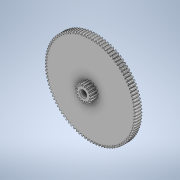
# Autodesk Inventor part: double_gear
Saved by Autodesk Inventor 2022.3 (Build 263350000, 350)
## iProperties
Created: 2022-06-10
Part Number: double_gear
Material: Generic
Document SubType Name: Modeling
Designer: Martijn
Density: 1 g/cm^3
Appearance: Default
Author: Martijn
Autodesk Inventor part; units mm, degrees
(part 1 of 3)
ref_plane "YZ Plane" through (0, 0, 0) normal (1, 0, 0) x (0, 1, 0)
ref_plane "XZ Plane" through (0, 0, 0) normal (0, 1, 0) x (-1, 0, 0)
ref_plane "XY Plane" through (0, 0, 0) normal (0, 0, 1) x (1, 0, 0)
sketch "Sketch1" plane through (0, 0, 0) normal (0, 0, 1) x (1, 0, 0)
  arc A0 (48.7229, -1.6254) -> (48.7288, -1.4372) centre (0, 0) ccw
  arc A1 (49.0225, -1.0633) -> (48.7288, -1.4372) centre (49.1286, -1.449) ccw
  spline S0 degree 3 poles (49.0225, -1.0633) (49.8054, -0.8336) (50.3699, -0.638) (50.9987, -0.3781) knots 0 0 0 0 1 1 1 1
  line L0 (49.0225, -1.0633) -> (49.8054, -0.8336) construction
  line L1 (49.8054, -0.8336) -> (50.3699, -0.638) construction
  line L2 (50.3699, -0.638) -> (50.9987, -0.3781) construction
  arc A2 (50.9987, -0.3781) -> (50.9987, 0.3781) centre (0, 0) ccw
  spline S1 degree 3 poles (50.9987, 0.3781) (50.3699, 0.638) (49.8054, 0.8336) (49.0225, 1.0633) knots 0 0 0 0 1 1 1 1
  line L3 (50.9987, 0.3781) -> (50.3699, 0.638) construction
  line L4 (50.3699, 0.638) -> (49.8054, 0.8336) construction
  line L5 (49.8054, 0.8336) -> (49.0225, 1.0633) construction
  arc A3 (48.7288, 1.4372) -> (49.0225, 1.0633) centre (49.1286, 1.449) ccw
  arc A4 (48.7288, 1.4372) -> (48.7229, 1.6254) centre (0, 0) ccw
  arc A5 (48.9926, 2.0169) -> (48.7229, 1.6254) centre (49.1227, 1.6387) ccw
  spline S2 degree 3 poles (48.9926, 2.0169) (49.7595, 2.2954) (50.3106, 2.526) (50.9218, 2.8249) knots 0 0 0 0 1 1 1 1
  line L6 (48.9926, 2.0169) -> (49.7595, 2.2954) construction
  line L7 (49.7595, 2.2954) -> (50.3106, 2.526) construction
  line L8 (50.3106, 2.526) -> (50.9218, 2.8249) construction
  arc A6 (50.9218, 2.8249) -> (50.8743, 3.5795) centre (0, 0) ccw
  spline S3 degree 3 poles (50.8743, 3.5795) (50.2305, 3.7995) (49.6548, 3.9592) (48.859, 4.1394) knots 0 0 0 0 1 1 1 1
  line L9 (50.8743, 3.5795) -> (50.2305, 3.7995) construction
  line L10 (50.2305, 3.7995) -> (49.6548, 3.9592) construction
  line L11 (49.6548, 3.9592) -> (48.859, 4.1394) construction
  arc A7 (48.5424, 4.4941) -> (48.859, 4.1394) centre (48.9407, 4.5309) ccw
  arc A8 (48.5424, 4.4941) -> (48.5247, 4.6815) centre (0, 0) ccw
  arc A9 (48.7692, 5.0892) -> (48.5247, 4.6815) centre (48.9228, 4.7199) ccw
  spline S4 degree 3 poles (48.7692, 5.0892) (49.5171, 5.4153) (50.0527, 5.68) (50.6439, 6.0168) knots 0 0 0 0 1 1 1 1
  line L12 (48.7692, 5.0892) -> (49.5171, 5.4153) construction
  line L13 (49.5171, 5.4153) -> (50.0527, 5.68) construction
  line L14 (50.0527, 5.68) -> (50.6439, 6.0168) construction
  arc A10 (50.6439, 6.0168) -> (50.5492, 6.7669) centre (0, 0) ccw
  spline S5 degree 3 poles (50.5492, 6.7669) (49.8928, 6.946) (49.3082, 7.0693) (48.5027, 7.1991) knots 0 0 0 0 1 1 1 1
  line L15 (50.5492, 6.7669) -> (49.8928, 6.946) construction
  line L16 (49.8928, 6.946) -> (49.3082, 7.0693) construction
  line L17 (49.3082, 7.0693) -> (48.5027, 7.1991) construction
  arc A11 (48.1644, 7.5332) -> (48.5027, 7.1991) centre (48.5596, 7.595) ccw
  arc A12 (48.1644, 7.5332) -> (48.135, 7.7191) centre (0, 0) ccw
  arc A13 (48.3535, 8.1414) -> (48.135, 7.7191) centre (48.5299, 7.7825) ccw
  spline S6 degree 3 poles (48.3535, 8.1414) (49.0794, 8.5138) (49.5973, 8.8117) (50.1662, 9.1848) knots 0 0 0 0 1 1 1 1
  line L18 (48.3535, 8.1414) -> (49.0794, 8.5138) construction
  line L19 (49.0794, 8.5138) -> (49.5973, 8.8117) construction
  line L20 (49.5973, 8.8117) -> (50.1662, 9.1848) construction
  arc A14 (50.1662, 9.1848) -> (50.0245, 9.9276) centre (0, 0) ccw
  spline S7 degree 3 poles (50.0245, 9.9276) (49.3582, 10.0651) (48.767, 10.1514) (47.955, 10.2304) knots 0 0 0 0 1 1 1 1
  line L21 (50.0245, 9.9276) -> (49.3582, 10.0651) construction
  line L22 (49.3582, 10.0651) -> (48.767, 10.1514) construction
  line L23 (48.767, 10.1514) -> (47.955, 10.2304) construction
  arc A15 (47.5964, 10.5426) -> (47.955, 10.2304) centre (47.9869, 10.6291) ccw
  arc A16 (47.5964, 10.5426) -> (47.5553, 10.7263) centre (0, 0) ccw
  arc A17 (47.7468, 11.1615) -> (47.5553, 10.7263) centre (47.9455, 10.8143) ccw
  spline S8 degree 3 poles (47.7468, 11.1615) (48.448, 11.5787) (48.9462, 11.9085) (49.4905, 12.3167) knots 0 0 0 0 1 1 1 1
  line L24 (47.7468, 11.1615) -> (48.448, 11.5787) construction
  line L25 (48.448, 11.5787) -> (48.9462, 11.9085) construction
  line L26 (48.9462, 11.9085) -> (49.4905, 12.3167) construction
  arc A18 (49.4905, 12.3167) -> (49.3024, 13.049) centre (0, 0) ccw
  spline S9 degree 3 poles (49.3024, 13.049) (48.6288, 13.1445) (48.0334, 13.1935) (47.218, 13.2213) knots 0 0 0 0 1 1 1 1
  line L27 (49.3024, 13.049) -> (48.6288, 13.1445) construction
  line L28 (48.6288, 13.1445) -> (48.0334, 13.1935) construction
  line L29 (48.0334, 13.1935) -> (47.218, 13.2213) construction
  arc A19 (46.8405, 13.5104) -> (47.218, 13.2213) centre (47.2248, 13.6213) ccw
  arc A20 (46.8405, 13.5104) -> (46.788, 13.6912) centre (0, 0) ccw
  arc A21 (46.9518, 14.1375) -> (46.788, 13.6912) centre (47.1719, 13.8035) ccw
  spline S10 degree 3 poles (46.9518, 14.1375) (47.6253, 14.5979) (48.1018, 14.9584) (48.6194, 15.3999) knots 0 0 0 0 1 1 1 1
  line L30 (46.9518, 14.1375) -> (47.6253, 14.5979) construction
  line L31 (47.6253, 14.5979) -> (48.1018, 14.9584) construction
  line L32 (48.1018, 14.9584) -> (48.6194, 15.3999) construction
  arc A22 (48.6194, 15.3999) -> (48.3858, 16.119) centre (0, 0) ccw
  spline S11 degree 3 poles (48.3858, 16.119) (47.7075, 16.172) (47.1102, 16.1835) (46.2946, 16.1601) knots 0 0 0 0 1 1 1 1
  line L33 (48.3858, 16.119) -> (47.7075, 16.172) construction
  line L34 (47.7075, 16.172) -> (47.1102, 16.1835) construction
  line L35 (47.1102, 16.1835) -> (46.2946, 16.1601) construction
  arc A23 (45.8997, 16.4249) -> (46.2946, 16.1601) centre (46.2763, 16.5596) ccw
  arc A24 (45.8997, 16.4249) -> (45.836, 16.602) centre (0, 0) ccw
  arc A25 (45.9714, 17.0578) -> (45.836, 16.602) centre (46.2121, 16.7382) ccw
  spline S12 degree 3 poles (45.9714, 17.0578) (46.6147, 17.5595) (47.0677, 17.9492) (47.5565, 18.4224) knots 0 0 0 0 1 1 1 1
  line L36 (45.9714, 17.0578) -> (46.6147, 17.5595) construction
  line L37 (46.6147, 17.5595) -> (47.0677, 17.9492) construction
  line L38 (47.0677, 17.9492) -> (47.5565, 18.4224) construction
  arc A26 (47.5565, 18.4224) -> (47.2782, 19.1254) centre (0, 0) ccw
  spline S13 degree 3 poles (47.2782, 19.1254) (46.5979, 19.1356) (46.001, 19.1096) (45.1886, 19.035) knots 0 0 0 0 1 1 1 1
  line L39 (47.2782, 19.1254) -> (46.5979, 19.1356) construction
  line L40 (46.5979, 19.1356) -> (46.001, 19.1096) construction
  line L41 (46.001, 19.1096) -> (45.1886, 19.035) construction
  arc A27 (44.7778, 19.2745) -> (45.1886, 19.035) centre (45.1452, 19.4327) ccw
  arc A28 (44.7778, 19.2745) -> (44.7031, 19.4473) centre (0, 0) ccw
  arc A29 (44.8097, 19.9107) -> (44.7031, 19.4473) centre (45.0699, 19.6069) ccw
  spline S14 degree 3 poles (44.8097, 19.9107) (45.4202, 20.4519) (45.8478, 20.8692) (46.3059, 21.3721) knots 0 0 0 0 1 1 1 1
  line L42 (44.8097, 19.9107) -> (45.4202, 20.4519) construction
  line L43 (45.4202, 20.4519) -> (45.8478, 20.8692) construction
  line L44 (45.8478, 20.8692) -> (46.3059, 21.3721) construction
  arc A30 (46.3059, 21.3721) -> (45.984, 22.0563) centre (0, 0) ccw
  spline S15 degree 3 poles (45.984, 22.0563) (45.3044, 22.0238) (44.7103, 21.9604) (43.9042, 21.8349) knots 0 0 0 0 1 1 1 1
  line L45 (45.984, 22.0563) -> (45.3044, 22.0238) construction
  line L46 (45.3044, 22.0238) -> (44.7103, 21.9604) construction
  line L47 (44.7103, 21.9604) -> (43.9042, 21.8349) construction
  arc A31 (43.4792, 22.0481) -> (43.9042, 21.8349) centre (43.836, 22.229) ccw
  arc A32 (43.4792, 22.0481) -> (43.3938, 22.2159) centre (0, 0) ccw
  arc A33 (43.471, 22.685) -> (43.3938, 22.2159) centre (43.7498, 22.3981) ccw
  spline S16 degree 3 poles (43.471, 22.685) (44.0464, 23.2635) (44.4469, 23.7068) (44.8726, 24.2375) knots 0 0 0 0 1 1 1 1
  line L48 (43.471, 22.685) -> (44.0464, 23.2635) construction
  line L49 (44.0464, 23.2635) -> (44.4469, 23.7068) construction
  line L50 (44.4469, 23.7068) -> (44.8726, 24.2375) construction
  arc A34 (44.8726, 24.2375) -> (44.5083, 24.9001) centre (0, 0) ccw
  spline S17 degree 3 poles (44.5083, 24.9001) (43.8322, 24.825) (43.2432, 24.7244) (42.4465, 24.5486) knots 0 0 0 0 1 1 1 1
  line L51 (44.5083, 24.9001) -> (43.8322, 24.825) construction
  line L52 (43.8322, 24.825) -> (43.2432, 24.7244) construction
  line L53 (43.2432, 24.7244) -> (42.4465, 24.5486) construction
  arc A35 (42.009, 24.7347) -> (42.4465, 24.5486) centre (42.3537, 24.9377) ccw
  arc A36 (42.009, 24.7347) -> (41.9132, 24.8967) centre (0, 0) ccw
  arc A37 (41.9609, 25.3698) -> (41.9132, 24.8967) centre (42.2571, 25.101) ccw
  spline S18 degree 3 poles (41.9609, 25.3698) (42.4987, 25.9832) (42.8706, 26.4509) (43.2622, 27.0072) knots 0 0 0 0 1 1 1 1
  line L54 (41.9609, 25.3698) -> (42.4987, 25.9832) construction
  line L55 (42.4987, 25.9832) -> (42.8706, 26.4509) construction
  line L56 (42.8706, 26.4509) -> (43.2622, 27.0072) construction
  arc A38 (43.2622, 27.0072) -> (42.857, 27.6457) centre (0, 0) ccw
  spline S19 degree 3 poles (42.857, 27.6457) (42.1869, 27.5283) (41.6054, 27.3909) (40.8213, 27.1654) knots 0 0 0 0 1 1 1 1
  line L57 (42.857, 27.6457) -> (42.1869, 27.5283) construction
  line L58 (42.1869, 27.5283) -> (41.6054, 27.3909) construction
  line L59 (41.6054, 27.3909) -> (40.8213, 27.1654) construction
  arc A39 (40.373, 27.3237) -> (40.8213, 27.1654) centre (40.7043, 27.5479) ccw
  arc A40 (40.373, 27.3237) -> (40.2672, 27.4794) centre (0, 0) ccw
  arc A41 (40.2851, 27.9545) -> (40.2672, 27.4794) centre (40.5976, 27.7048) ccw
  spline S20 degree 3 poles (40.2851, 27.9545) (40.7834, 28.6005) (41.1252, 29.0905) (41.481, 29.6704) knots 0 0 0 0 1 1 1 1
  line L60 (40.2851, 27.9545) -> (40.7834, 28.6005) construction
  line L61 (40.7834, 28.6005) -> (41.1252, 29.0905) construction
  line L62 (41.1252, 29.0905) -> (41.481, 29.6704) construction
  arc A42 (41.481, 29.6704) -> (41.0366, 30.2821) centre (0, 0) ccw
  spline S21 degree 3 poles (41.0366, 30.2821) (40.3751, 30.1229) (39.8034, 29.9493) (39.0351, 29.675) knots 0 0 0 0 1 1 1 1
  line L63 (41.0366, 30.2821) -> (40.3751, 30.1229) construction
  line L64 (40.3751, 30.1229) -> (39.8034, 29.9493) construction
  line L65 (39.8034, 29.9493) -> (39.0351, 29.675) construction
  arc A43 (38.5777, 29.8048) -> (39.0351, 29.675) centre (38.8942, 30.0493) ccw
  arc A44 (38.5777, 29.8048) -> (38.4623, 29.9535) centre (0, 0) ccw
  arc A45 (38.4503, 30.4288) -> (38.4623, 29.9535) centre (38.7779, 30.1993) ccw
  spline S22 degree 3 poles (38.4503, 30.4288) (38.9071, 31.1049) (39.2174, 31.6154) (39.5361, 32.2165) knots 0 0 0 0 1 1 1 1
  line L66 (38.4503, 30.4288) -> (38.9071, 31.1049) construction
  line L67 (38.9071, 31.1049) -> (39.2174, 31.6154) construction
  line L68 (39.2174, 31.6154) -> (39.5361, 32.2165) construction
  arc A46 (39.5361, 32.2165) -> (39.0542, 32.7991) centre (0, 0) ccw
  spline S23 degree 3 poles (39.0542, 32.7991) (38.404, 32.5986) (37.8444, 32.3894) (37.0947, 32.0674) knots 0 0 0 0 1 1 1 1
  line L69 (39.0542, 32.7991) -> (38.404, 32.5986) construction
  line L70 (38.404, 32.5986) -> (37.8444, 32.3894) construction
  line L71 (37.8444, 32.3894) -> (37.0947, 32.0674) construction
  arc A47 (36.6301, 32.1683) -> (37.0947, 32.0674) centre (36.9306, 32.4322) ccw
  arc A48 (36.6301, 32.1683) -> (36.5056, 32.3095) centre (0, 0) ccw
  arc A49 (36.4638, 32.7831) -> (36.5056, 32.3095) centre (36.8051, 32.5746) ccw
  spline S24 degree 3 poles (36.4638, 32.7831) (36.8772, 33.4865) (37.1549, 34.0155) (37.4352, 34.6354) knots 0 0 0 0 1 1 1 1
  line L72 (36.4638, 32.7831) -> (36.8772, 33.4865) construction
  line L73 (36.8772, 33.4865) -> (37.1549, 34.0155) construction
  line L74 (37.1549, 34.0155) -> (37.4352, 34.6354) construction
  arc A50 (37.4352, 34.6354) -> (36.9176, 35.1866) centre (0, 0) ccw
  spline S25 degree 3 poles (36.9176, 35.1866) (36.2814, 34.9457) (35.7359, 34.7018) (35.008, 34.3334) knots 0 0 0 0 1 1 1 1
  line L75 (36.9176, 35.1866) -> (36.2814, 34.9457) construction
  line L76 (36.2814, 34.9457) -> (35.7359, 34.7018) construction
  line L77 (35.7359, 34.7018) -> (35.008, 34.3334) construction
  arc A51 (34.538, 34.4048) -> (35.008, 34.3334) centre (34.8213, 34.6871) ccw
  arc A52 (34.538, 34.4048) -> (34.4048, 34.538) centre (0, 0) ccw
  arc A53 (34.3334, 35.008) -> (34.4048, 34.538) centre (34.6871, 34.8213) ccw
  spline S26 degree 3 poles (34.3334, 35.008) (34.7018, 35.7359) (34.9457, 36.2814) (35.1866, 36.9176) knots 0 0 0 0 1 1 1 1
  line L78 (34.3334, 35.008) -> (34.7018, 35.7359) construction
  line L79 (34.7018, 35.7359) -> (34.9457, 36.2814) construction
  line L80 (34.9457, 36.2814) -> (35.1866, 36.9176) construction
  arc A54 (35.1866, 36.9176) -> (34.6354, 37.4352) centre (0, 0) ccw
  spline S27 degree 3 poles (34.6354, 37.4352) (34.0155, 37.1549) (33.4865, 36.8772) (32.7831, 36.4638) knots 0 0 0 0 1 1 1 1
  line L81 (34.6354, 37.4352) -> (34.0155, 37.1549) construction
  line L82 (34.0155, 37.1549) -> (33.4865, 36.8772) construction
  line L83 (33.4865, 36.8772) -> (32.7831, 36.4638) construction
  arc A55 (32.3095, 36.5056) -> (32.7831, 36.4638) centre (32.5746, 36.8051) ccw
  arc A56 (32.3095, 36.5056) -> (32.1683, 36.6301) centre (0, 0) ccw
  arc A57 (32.0674, 37.0947) -> (32.1683, 36.6301) centre (32.4322, 36.9306) ccw
  spline S28 degree 3 poles (32.0674, 37.0947) (32.3894, 37.8444) (32.5986, 38.404) (32.7991, 39.0542) knots 0 0 0 0 1 1 1 1
  line L84 (32.0674, 37.0947) -> (32.3894, 37.8444) construction
  line L85 (32.3894, 37.8444) -> (32.5986, 38.404) construction
  line L86 (32.5986, 38.404) -> (32.7991, 39.0542) construction
  arc A58 (32.7991, 39.0542) -> (32.2165, 39.5361) centre (0, 0) ccw
  spline S29 degree 3 poles (32.2165, 39.5361) (31.6154, 39.2174) (31.1049, 38.9071) (30.4288, 38.4503) knots 0 0 0 0 1 1 1 1
  line L87 (32.2165, 39.5361) -> (31.6154, 39.2174) construction
  line L88 (31.6154, 39.2174) -> (31.1049, 38.9071) construction
  line L89 (31.1049, 38.9071) -> (30.4288, 38.4503) construction
  arc A59 (29.9535, 38.4623) -> (30.4288, 38.4503) centre (30.1993, 38.7779) ccw
  arc A60 (29.9535, 38.4623) -> (29.8048, 38.5777) centre (0, 0) ccw
  arc A61 (29.675, 39.0351) -> (29.8048, 38.5777) centre (30.0493, 38.8942) ccw
  spline S30 degree 3 poles (29.675, 39.0351) (29.9493, 39.8034) (30.1229, 40.3751) (30.2821, 41.0366) knots 0 0 0 0 1 1 1 1
  line L90 (29.675, 39.0351) -> (29.9493, 39.8034) construction
  line L91 (29.9493, 39.8034) -> (30.1229, 40.3751) construction
  line L92 (30.1229, 40.3751) -> (30.2821, 41.0366) construction
  arc A62 (30.2821, 41.0366) -> (29.6704, 41.481) centre (0, 0) ccw
  spline S31 degree 3 poles (29.6704, 41.481) (29.0905, 41.1252) (28.6005, 40.7834) (27.9545, 40.2851) knots 0 0 0 0 1 1 1 1
  line L93 (29.6704, 41.481) -> (29.0905, 41.1252) construction
  line L94 (29.0905, 41.1252) -> (28.6005, 40.7834) construction
  line L95 (28.6005, 40.7834) -> (27.9545, 40.2851) construction
  arc A63 (27.4794, 40.2672) -> (27.9545, 40.2851) centre (27.7048, 40.5976) ccw
  arc A64 (27.4794, 40.2672) -> (27.3237, 40.373) centre (0, 0) ccw
  arc A65 (27.1654, 40.8213) -> (27.3237, 40.373) centre (27.5479, 40.7043) ccw
  spline S32 degree 3 poles (27.1654, 40.8213) (27.3909, 41.6054) (27.5283, 42.1869) (27.6457, 42.857) knots 0 0 0 0 1 1 1 1
  line L96 (27.1654, 40.8213) -> (27.3909, 41.6054) construction
  line L97 (27.3909, 41.6054) -> (27.5283, 42.1869) construction
  line L98 (27.5283, 42.1869) -> (27.6457, 42.857) construction
  arc A66 (27.6457, 42.857) -> (27.0072, 43.2622) centre (0, 0) ccw
  spline S33 degree 3 poles (27.0072, 43.2622) (26.4509, 42.8706) (25.9832, 42.4987) (25.3698, 41.9609) knots 0 0 0 0 1 1 1 1
  line L99 (27.0072, 43.2622) -> (26.4509, 42.8706) construction
  line L100 (26.4509, 42.8706) -> (25.9832, 42.4987) construction
  line L101 (25.9832, 42.4987) -> (25.3698, 41.9609) construction
  arc A67 (24.8967, 41.9132) -> (25.3698, 41.9609) centre (25.101, 42.2571) ccw
  arc A68 (24.8967, 41.9132) -> (24.7347, 42.009) centre (0, 0) ccw
  arc A69 (24.5486, 42.4465) -> (24.7347, 42.009) centre (24.9377, 42.3537) ccw
  spline S34 degree 3 poles (24.5486, 42.4465) (24.7244, 43.2432) (24.825, 43.8322) (24.9001, 44.5083) knots 0 0 0 0 1 1 1 1
  line L102 (24.5486, 42.4465) -> (24.7244, 43.2432) construction
  line L103 (24.7244, 43.2432) -> (24.825, 43.8322) construction
  line L104 (24.825, 43.8322) -> (24.9001, 44.5083) construction
  arc A70 (24.9001, 44.5083) -> (24.2375, 44.8726) centre (0, 0) ccw
  spline S35 degree 3 poles (24.2375, 44.8726) (23.7068, 44.4469) (23.2635, 44.0464) (22.685, 43.471) knots 0 0 0 0 1 1 1 1
  line L105 (24.2375, 44.8726) -> (23.7068, 44.4469) construction
  line L106 (23.7068, 44.4469) -> (23.2635, 44.0464) construction
  line L107 (23.2635, 44.0464) -> (22.685, 43.471) construction
  arc A71 (22.2159, 43.3938) -> (22.685, 43.471) centre (22.3981, 43.7498) ccw
  arc A72 (22.2159, 43.3938) -> (22.0481, 43.4792) centre (0, 0) ccw
  arc A73 (21.8349, 43.9042) -> (22.0481, 43.4792) centre (22.229, 43.836) ccw
  spline S36 degree 3 poles (21.8349, 43.9042) (21.9604, 44.7103) (22.0238, 45.3044) (22.0563, 45.984) knots 0 0 0 0 1 1 1 1
  line L108 (21.8349, 43.9042) -> (21.9604, 44.7103) construction
  line L109 (21.9604, 44.7103) -> (22.0238, 45.3044) construction
  line L110 (22.0238, 45.3044) -> (22.0563, 45.984) construction
  arc A74 (22.0563, 45.984) -> (21.3721, 46.3059) centre (0, 0) ccw
  spline S37 degree 3 poles (21.3721, 46.3059) (20.8692, 45.8478) (20.4519, 45.4202) (19.9107, 44.8097) knots 0 0 0 0 1 1 1 1
  line L111 (21.3721, 46.3059) -> (20.8692, 45.8478) construction
  line L112 (20.8692, 45.8478) -> (20.4519, 45.4202) construction
  line L113 (20.4519, 45.4202) -> (19.9107, 44.8097) construction
  arc A75 (19.4473, 44.7031) -> (19.9107, 44.8097) centre (19.6069, 45.0699) ccw
  arc A76 (19.4473, 44.7031) -> (19.2745, 44.7778) centre (0, 0) ccw
  arc A77 (19.035, 45.1886) -> (19.2745, 44.7778) centre (19.4327, 45.1452) ccw
  spline S38 degree 3 poles (19.035, 45.1886) (19.1096, 46.001) (19.1356, 46.5979) (19.1254, 47.2782) knots 0 0 0 0 1 1 1 1
  line L114 (19.035, 45.1886) -> (19.1096, 46.001) construction
  line L115 (19.1096, 46.001) -> (19.1356, 46.5979) construction
  line L116 (19.1356, 46.5979) -> (19.1254, 47.2782) construction
  arc A78 (19.1254, 47.2782) -> (18.4224, 47.5565) centre (0, 0) ccw
  spline S39 degree 3 poles (18.4224, 47.5565) (17.9492, 47.0677) (17.5595, 46.6147) (17.0578, 45.9714) knots 0 0 0 0 1 1 1 1
  line L117 (18.4224, 47.5565) -> (17.9492, 47.0677) construction
  line L118 (17.9492, 47.0677) -> (17.5595, 46.6147) construction
  line L119 (17.5595, 46.6147) -> (17.0578, 45.9714) construction
  arc A79 (16.602, 45.836) -> (17.0578, 45.9714) centre (16.7382, 46.2121) ccw
  arc A80 (16.602, 45.836) -> (16.4249, 45.8997) centre (0, 0) ccw
  arc A81 (16.1601, 46.2946) -> (16.4249, 45.8997) centre (16.5596, 46.2763) ccw
  spline S40 degree 3 poles (16.1601, 46.2946) (16.1835, 47.1102) (16.172, 47.7075) (16.119, 48.3858) knots 0 0 0 0 1 1 1 1
  line L120 (16.1601, 46.2946) -> (16.1835, 47.1102) construction
  line L121 (16.1835, 47.1102) -> (16.172, 47.7075) construction
  line L122 (16.172, 47.7075) -> (16.119, 48.3858) construction
  arc A82 (16.119, 48.3858) -> (15.3999, 48.6194) centre (0, 0) ccw
  spline S41 degree 3 poles (15.3999, 48.6194) (14.9584, 48.1018) (14.5979, 47.6253) (14.1375, 46.9518) knots 0 0 0 0 1 1 1 1
  line L123 (15.3999, 48.6194) -> (14.9584, 48.1018) construction
  line L124 (14.9584, 48.1018) -> (14.5979, 47.6253) construction
  line L125 (14.5979, 47.6253) -> (14.1375, 46.9518) construction
  arc A83 (13.6912, 46.788) -> (14.1375, 46.9518) centre (13.8035, 47.1719) ccw
  arc A84 (13.6912, 46.788) -> (13.5104, 46.8405) centre (0, 0) ccw
  arc A85 (13.2213, 47.218) -> (13.5104, 46.8405) centre (13.6213, 47.2248) ccw
  spline S42 degree 3 poles (13.2213, 47.218) (13.1935, 48.0334) (13.1445, 48.6288) (13.049, 49.3024) knots 0 0 0 0 1 1 1 1
  line L126 (13.2213, 47.218) -> (13.1935, 48.0334) construction
  line L127 (13.1935, 48.0334) -> (13.1445, 48.6288) construction
  line L128 (13.1445, 48.6288) -> (13.049, 49.3024) construction
  arc A86 (13.049, 49.3024) -> (12.3167, 49.4905) centre (0, 0) ccw
  spline S43 degree 3 poles (12.3167, 49.4905) (11.9085, 48.9462) (11.5787, 48.448) (11.1615, 47.7468) knots 0 0 0 0 1 1 1 1
  line L129 (12.3167, 49.4905) -> (11.9085, 48.9462) construction
  line L130 (11.9085, 48.9462) -> (11.5787, 48.448) construction
  line L131 (11.5787, 48.448) -> (11.1615, 47.7468) construction
  arc A87 (10.7263, 47.5553) -> (11.1615, 47.7468) centre (10.8143, 47.9455) ccw
  arc A88 (10.7263, 47.5553) -> (10.5426, 47.5964) centre (0, 0) ccw
  arc A89 (10.2304, 47.955) -> (10.5426, 47.5964) centre (10.6291, 47.9869) ccw
  spline S44 degree 3 poles (10.2304, 47.955) (10.1514, 48.767) (10.0651, 49.3582) (9.9276, 50.0245) knots 0 0 0 0 1 1 1 1
  line L132 (10.2304, 47.955) -> (10.1514, 48.767) construction
  line L133 (10.1514, 48.767) -> (10.0651, 49.3582) construction
  line L134 (10.0651, 49.3582) -> (9.9276, 50.0245) construction
  arc A90 (9.9276, 50.0245) -> (9.1848, 50.1662) centre (0, 0) ccw
  spline S45 degree 3 poles (9.1848, 50.1662) (8.8117, 49.5973) (8.5138, 49.0794) (8.1414, 48.3535) knots 0 0 0 0 1 1 1 1
  line L135 (9.1848, 50.1662) -> (8.8117, 49.5973) construction
  line L136 (8.8117, 49.5973) -> (8.5138, 49.0794) construction
  line L137 (8.5138, 49.0794) -> (8.1414, 48.3535) construction
  arc A91 (7.7191, 48.135) -> (8.1414, 48.3535) centre (7.7825, 48.5299) ccw
  arc A92 (7.7191, 48.135) -> (7.5332, 48.1644) centre (0, 0) ccw
  arc A93 (7.1991, 48.5027) -> (7.5332, 48.1644) centre (7.595, 48.5596) ccw
  spline S46 degree 3 poles (7.1991, 48.5027) (7.0693, 49.3082) (6.946, 49.8928) (6.7669, 50.5492) knots 0 0 0 0 1 1 1 1
  line L138 (7.1991, 48.5027) -> (7.0693, 49.3082) construction
  line L139 (7.0693, 49.3082) -> (6.946, 49.8928) construction
  line L140 (6.946, 49.8928) -> (6.7669, 50.5492) construction
  arc A94 (6.7669, 50.5492) -> (6.0168, 50.6439) centre (0, 0) ccw
  spline S47 degree 3 poles (6.0168, 50.6439) (5.68, 50.0527) (5.4153, 49.5171) (5.0892, 48.7692) knots 0 0 0 0 1 1 1 1
  line L141 (6.0168, 50.6439) -> (5.68, 50.0527) construction
  line L142 (5.68, 50.0527) -> (5.4153, 49.5171) construction
  line L143 (5.4153, 49.5171) -> (5.0892, 48.7692) construction
  arc A95 (4.6815, 48.5247) -> (5.0892, 48.7692) centre (4.7199, 48.9228) ccw
  arc A96 (4.6815, 48.5247) -> (4.4941, 48.5424) centre (0, 0) ccw
  arc A97 (4.1394, 48.859) -> (4.4941, 48.5424) centre (4.5309, 48.9407) ccw
  spline S48 degree 3 poles (4.1394, 48.859) (3.9592, 49.6548) (3.7995, 50.2305) (3.5795, 50.8743) knots 0 0 0 0 1 1 1 1
  line L144 (4.1394, 48.859) -> (3.9592, 49.6548) construction
  line L145 (3.9592, 49.6548) -> (3.7995, 50.2305) construction
  line L146 (3.7995, 50.2305) -> (3.5795, 50.8743) construction
  arc A98 (3.5795, 50.8743) -> (2.8249, 50.9218) centre (0, 0) ccw
  spline S49 degree 3 poles (2.8249, 50.9218) (2.526, 50.3106) (2.2954, 49.7595) (2.0169, 48.9926) knots 0 0 0 0 1 1 1 1
  line L147 (2.8249, 50.9218) -> (2.526, 50.3106) construction
  line L148 (2.526, 50.3106) -> (2.2954, 49.7595) construction
  line L149 (2.2954, 49.7595) -> (2.0169, 48.9926) construction
  arc A99 (1.6254, 48.7229) -> (2.0169, 48.9926) centre (1.6387, 49.1227) ccw
  arc A100 (1.6254, 48.7229) -> (1.4372, 48.7288) centre (0, 0) ccw
  arc A101 (1.0633, 49.0225) -> (1.4372, 48.7288) centre (1.449, 49.1286) ccw
  spline S50 degree 3 poles (1.0633, 49.0225) (0.8336, 49.8054) (0.638, 50.3699) (0.3781, 50.9987) knots 0 0 0 0 1 1 1 1
  line L150 (1.0633, 49.0225) -> (0.8336, 49.8054) construction
  line L151 (0.8336, 49.8054) -> (0.638, 50.3699) construction
  line L152 (0.638, 50.3699) -> (0.3781, 50.9987) construction
  arc A102 (0.3781, 50.9987) -> (-0.3781, 50.9987) centre (0, 0) ccw
  spline S51 degree 3 poles (-0.3781, 50.9987) (-0.638, 50.3699) (-0.8336, 49.8054) (-1.0633, 49.0225) knots 0 0 0 0 1 1 1 1
  line L153 (-0.3781, 50.9987) -> (-0.638, 50.3699) construction
  line L154 (-0.638, 50.3699) -> (-0.8336, 49.8054) construction
  line L155 (-0.8336, 49.8054) -> (-1.0633, 49.0225) construction
  arc A103 (-1.4372, 48.7288) -> (-1.0633, 49.0225) centre (-1.449, 49.1286) ccw
  arc A104 (-1.4372, 48.7288) -> (-1.6254, 48.7229) centre (0, 0) ccw
  arc A105 (-2.0169, 48.9926) -> (-1.6254, 48.7229) centre (-1.6387, 49.1227) ccw
  spline S52 degree 3 poles (-2.0169, 48.9926) (-2.2954, 49.7595) (-2.526, 50.3106) (-2.8249, 50.9218) knots 0 0 0 0 1 1 1 1
  line L156 (-2.0169, 48.9926) -> (-2.2954, 49.7595) construction
  line L157 (-2.2954, 49.7595) -> (-2.526, 50.3106) construction
  line L158 (-2.526, 50.3106) -> (-2.8249, 50.9218) construction
  arc A106 (-2.8249, 50.9218) -> (-3.5795, 50.8743) centre (0, 0) ccw
  spline S53 degree 3 poles (-3.5795, 50.8743) (-3.7995, 50.2305) (-3.9592, 49.6548) (-4.1394, 48.859) knots 0 0 0 0 1 1 1 1
  line L159 (-3.5795, 50.8743) -> (-3.7995, 50.2305) construction
  line L160 (-3.7995, 50.2305) -> (-3.9592, 49.6548) construction
  line L161 (-3.9592, 49.6548) -> (-4.1394, 48.859) construction
  arc A107 (-4.4941, 48.5424) -> (-4.1394, 48.859) centre (-4.5309, 48.9407) ccw
  arc A108 (-4.4941, 48.5424) -> (-4.6815, 48.5247) centre (0, 0) ccw
  arc A109 (-5.0892, 48.7692) -> (-4.6815, 48.5247) centre (-4.7199, 48.9228) ccw
  spline S54 degree 3 poles (-5.0892, 48.7692) (-5.4153, 49.5171) (-5.68, 50.0527) (-6.0168, 50.6439) knots 0 0 0 0 1 1 1 1
  line L162 (-5.0892, 48.7692) -> (-5.4153, 49.5171) construction
  line L163 (-5.4153, 49.5171) -> (-5.68, 50.0527) construction
  line L164 (-5.68, 50.0527) -> (-6.0168, 50.6439) construction
  arc A110 (-6.0168, 50.6439) -> (-6.7669, 50.5492) centre (0, 0) ccw
  spline S55 degree 3 poles (-6.7669, 50.5492) (-6.946, 49.8928) (-7.0693, 49.3082) (-7.1991, 48.5027) knots 0 0 0 0 1 1 1 1
  line L165 (-6.7669, 50.5492) -> (-6.946, 49.8928) construction
  line L166 (-6.946, 49.8928) -> (-7.0693, 49.3082) construction
  line L167 (-7.0693, 49.3082) -> (-7.1991, 48.5027) construction
  arc A111 (-7.5332, 48.1644) -> (-7.1991, 48.5027) centre (-7.595, 48.5596) ccw
  arc A112 (-7.5332, 48.1644) -> (-7.7191, 48.135) centre (0, 0) ccw
  arc A113 (-8.1414, 48.3535) -> (-7.7191, 48.135) centre (-7.7825, 48.5299) ccw
  spline S56 degree 3 poles (-8.1414, 48.3535) (-8.5138, 49.0794) (-8.8117, 49.5973) (-9.1848, 50.1662) knots 0 0 0 0 1 1 1 1
  line L168 (-8.1414, 48.3535) -> (-8.5138, 49.0794) construction
  line L169 (-8.5138, 49.0794) -> (-8.8117, 49.5973) construction
  line L170 (-8.8117, 49.5973) -> (-9.1848, 50.1662) construction
  arc A114 (-9.1848, 50.1662) -> (-9.9276, 50.0245) centre (0, 0) ccw
  spline S57 degree 3 poles (-9.9276, 50.0245) (-10.0651, 49.3582) (-10.1514, 48.767) (-10.2304, 47.955) knots 0 0 0 0 1 1 1 1
  line L171 (-9.9276, 50.0245) -> (-10.0651, 49.3582) construction
  line L172 (-10.0651, 49.3582) -> (-10.1514, 48.767) construction
  line L173 (-10.1514, 48.767) -> (-10.2304, 47.955) construction
  arc A115 (-10.5426, 47.5964) -> (-10.2304, 47.955) centre (-10.6291, 47.9869) ccw
  arc A116 (-10.5426, 47.5964) -> (-10.7263, 47.5553) centre (0, 0) ccw
  arc A117 (-11.1615, 47.7468) -> (-10.7263, 47.5553) centre (-10.8143, 47.9455) ccw
  spline S58 degree 3 poles (-11.1615, 47.7468) (-11.5787, 48.448) (-11.9085, 48.9462) (-12.3167, 49.4905) knots 0 0 0 0 1 1 1 1
  line L174 (-11.1615, 47.7468) -> (-11.5787, 48.448) construction
  line L175 (-11.5787, 48.448) -> (-11.9085, 48.9462) construction
  line L176 (-11.9085, 48.9462) -> (-12.3167, 49.4905) construction
  arc A118 (-12.3167, 49.4905) -> (-13.049, 49.3024) centre (0, 0) ccw
  spline S59 degree 3 poles (-13.049, 49.3024) (-13.1445, 48.6288) (-13.1935, 48.0334) (-13.2213, 47.218) knots 0 0 0 0 1 1 1 1
  line L177 (-13.049, 49.3024) -> (-13.1445, 48.6288) construction
  line L178 (-13.1445, 48.6288) -> (-13.1935, 48.0334) construction
  line L179 (-13.1935, 48.0334) -> (-13.2213, 47.218) construction
  arc A119 (-13.5104, 46.8405) -> (-13.2213, 47.218) centre (-13.6213, 47.2248) ccw
  arc A120 (-13.5104, 46.8405) -> (-13.6912, 46.788) centre (0, 0) ccw
  arc A121 (-14.1375, 46.9518) -> (-13.6912, 46.788) centre (-13.8035, 47.1719) ccw
  spline S60 degree 3 poles (-14.1375, 46.9518) (-14.5979, 47.6253) (-14.9584, 48.1018) (-15.3999, 48.6194) knots 0 0 0 0 1 1 1 1
  line L180 (-14.1375, 46.9518) -> (-14.5979, 47.6253) construction
  line L181 (-14.5979, 47.6253) -> (-14.9584, 48.1018) construction
  line L182 (-14.9584, 48.1018) -> (-15.3999, 48.6194) construction
  arc A122 (-15.3999, 48.6194) -> (-16.119, 48.3858) centre (0, 0) ccw
  spline S61 degree 3 poles (-16.119, 48.3858) (-16.172, 47.7075) (-16.1835, 47.1102) (-16.1601, 46.2946) knots 0 0 0 0 1 1 1 1
  line L183 (-16.119, 48.3858) -> (-16.172, 47.7075) construction
  line L184 (-16.172, 47.7075) -> (-16.1835, 47.1102) construction
  line L185 (-16.1835, 47.1102) -> (-16.1601, 46.2946) construction
  arc A123 (-16.4249, 45.8997) -> (-16.1601, 46.2946) centre (-16.5596, 46.2763) ccw
  arc A124 (-16.4249, 45.8997) -> (-16.602, 45.836) centre (0, 0) ccw
  arc A125 (-17.0578, 45.9714) -> (-16.602, 45.836) centre (-16.7382, 46.2121) ccw
  spline S62 degree 3 poles (-17.0578, 45.9714) (-17.5595, 46.6147) (-17.9492, 47.0677) (-18.4224, 47.5565) knots 0 0 0 0 1 1 1 1
  line L186 (-17.0578, 45.9714) -> (-17.5595, 46.6147) construction
  line L187 (-17.5595, 46.6147) -> (-17.9492, 47.0677) construction
  line L188 (-17.9492, 47.0677) -> (-18.4224, 47.5565) construction
  arc A126 (-18.4224, 47.5565) -> (-19.1254, 47.2782) centre (0, 0) ccw
  spline S63 degree 3 poles (-19.1254, 47.2782) (-19.1356, 46.5979) (-19.1096, 46.001) (-19.035, 45.1886) knots 0 0 0 0 1 1 1 1
  line L189 (-19.1254, 47.2782) -> (-19.1356, 46.5979) construction
  line L190 (-19.1356, 46.5979) -> (-19.1096, 46.001) construction
  line L191 (-19.1096, 46.001) -> (-19.035, 45.1886) construction
  arc A127 (-19.2745, 44.7778) -> (-19.035, 45.1886) centre (-19.4327, 45.1452) ccw
  arc A128 (-19.2745, 44.7778) -> (-19.4473, 44.7031) centre (0, 0) ccw
  arc A129 (-19.9107, 44.8097) -> (-19.4473, 44.7031) centre (-19.6069, 45.0699) ccw
  spline S64 degree 3 poles (-19.9107, 44.8097) (-20.4519, 45.4202) (-20.8692, 45.8478) (-21.3721, 46.3059) knots 0 0 0 0 1 1 1 1
  line L192 (-19.9107, 44.8097) -> (-20.4519, 45.4202) construction
  line L193 (-20.4519, 45.4202) -> (-20.8692, 45.8478) construction
  line L194 (-20.8692, 45.8478) -> (-21.3721, 46.3059) construction
  arc A130 (-21.3721, 46.3059) -> (-22.0563, 45.984) centre (0, 0) ccw
  spline S65 degree 3 poles (-22.0563, 45.984) (-22.0238, 45.3044) (-21.9604, 44.7103) (-21.8349, 43.9042) knots 0 0 0 0 1 1 1 1
  line L195 (-22.0563, 45.984) -> (-22.0238, 45.3044) construction
  line L196 (-22.0238, 45.3044) -> (-21.9604, 44.7103) construction
  line L197 (-21.9604, 44.7103) -> (-21.8349, 43.9042) construction
  arc A131 (-22.0481, 43.4792) -> (-21.8349, 43.9042) centre (-22.229, 43.836) ccw
  arc A132 (-22.0481, 43.4792) -> (-22.2159, 43.3938) centre (0, 0) ccw
  arc A133 (-22.685, 43.471) -> (-22.2159, 43.3938) centre (-22.3981, 43.7498) ccw
  spline S66 degree 3 poles (-22.685, 43.471) (-23.2635, 44.0464) (-23.7068, 44.4469) (-24.2375, 44.8726) knots 0 0 0 0 1 1 1 1
  line L198 (-22.685, 43.471) -> (-23.2635, 44.0464) construction
  line L199 (-23.2635, 44.0464) -> (-23.7068, 44.4469) construction
  line L200 (-23.7068, 44.4469) -> (-24.2375, 44.8726) construction
  arc A134 (-24.2375, 44.8726) -> (-24.9001, 44.5083) centre (0, 0) ccw
  spline S67 degree 3 poles (-24.9001, 44.5083) (-24.825, 43.8322) (-24.7244, 43.2432) (-24.5486, 42.4465) knots 0 0 0 0 1 1 1 1
  line L201 (-24.9001, 44.5083) -> (-24.825, 43.8322) construction
  line L202 (-24.825, 43.8322) -> (-24.7244, 43.2432) construction
  line L203 (-24.7244, 43.2432) -> (-24.5486, 42.4465) construction
  arc A135 (-24.7347, 42.009) -> (-24.5486, 42.4465) centre (-24.9377, 42.3537) ccw
  arc A136 (-24.7347, 42.009) -> (-24.8967, 41.9132) centre (0, 0) ccw
  arc A137 (-25.3698, 41.9609) -> (-24.8967, 41.9132) centre (-25.101, 42.2571) ccw
  spline S68 degree 3 poles (-25.3698, 41.9609) (-25.9832, 42.4987) (-26.4509, 42.8706) (-27.0072, 43.2622) knots 0 0 0 0 1 1 1 1
  line L204 (-25.3698, 41.9609) -> (-25.9832, 42.4987) construction
  line L205 (-25.9832, 42.4987) -> (-26.4509, 42.8706) construction
  line L206 (-26.4509, 42.8706) -> (-27.0072, 43.2622) construction
  arc A138 (-27.0072, 43.2622) -> (-27.6457, 42.857) centre (0, 0) ccw
  spline S69 degree 3 poles (-27.6457, 42.857) (-27.5283, 42.1869) (-27.3909, 41.6054) (-27.1654, 40.8213) knots 0 0 0 0 1 1 1 1
  line L207 (-27.6457, 42.857) -> (-27.5283, 42.1869) construction
  line L208 (-27.5283, 42.1869) -> (-27.3909, 41.6054) construction
  line L209 (-27.3909, 41.6054) -> (-27.1654, 40.8213) construction
  arc A139 (-27.3237, 40.373) -> (-27.1654, 40.8213) centre (-27.5479, 40.7043) ccw
  arc A140 (-27.3237, 40.373) -> (-27.4794, 40.2672) centre (0, 0) ccw
  arc A141 (-27.9545, 40.2851) -> (-27.4794, 40.2672) centre (-27.7048, 40.5976) ccw
  spline S70 degree 3 poles (-27.9545, 40.2851) (-28.6005, 40.7834) (-29.0905, 41.1252) (-29.6704, 41.481) knots 0 0 0 0 1 1 1 1
  line L210 (-27.9545, 40.2851) -> (-28.6005, 40.7834) construction
  line L211 (-28.6005, 40.7834) -> (-29.0905, 41.1252) construction
  line L212 (-29.0905, 41.1252) -> (-29.6704, 41.481) construction
  arc A142 (-29.6704, 41.481) -> (-30.2821, 41.0366) centre (0, 0) ccw
  spline S71 degree 3 poles (-30.2821, 41.0366) (-30.1229, 40.3751) (-29.9493, 39.8034) (-29.675, 39.0351) knots 0 0 0 0 1 1 1 1
  line L213 (-30.2821, 41.0366) -> (-30.1229, 40.3751) construction
  line L214 (-30.1229, 40.3751) -> (-29.9493, 39.8034) construction
  line L215 (-29.9493, 39.8034) -> (-29.675, 39.0351) construction
  arc A143 (-29.8048, 38.5777) -> (-29.675, 39.0351) centre (-30.0493, 38.8942) ccw
  arc A144 (-29.8048, 38.5777) -> (-29.9535, 38.4623) centre (0, 0) ccw
  arc A145 (-30.4288, 38.4503) -> (-29.9535, 38.4623) centre (-30.1993, 38.7779) ccw
  spline S72 degree 3 poles (-30.4288, 38.4503) (-31.1049, 38.9071) (-31.6154, 39.2174) (-32.2165, 39.5361) knots 0 0 0 0 1 1 1 1
  line L216 (-30.4288, 38.4503) -> (-31.1049, 38.9071) construction
  line L217 (-31.1049, 38.9071) -> (-31.6154, 39.2174) construction
  line L218 (-31.6154, 39.2174) -> (-32.2165, 39.5361) construction
  arc A146 (-32.2165, 39.5361) -> (-32.7991, 39.0542) centre (0, 0) ccw
  spline S73 degree 3 poles (-32.7991, 39.0542) (-32.5986, 38.404) (-32.3894, 37.8444) (-32.0674, 37.0947) knots 0 0 0 0 1 1 1 1
  line L219 (-32.7991, 39.0542) -> (-32.5986, 38.404) construction
  line L220 (-32.5986, 38.404) -> (-32.3894, 37.8444) construction
  line L221 (-32.3894, 37.8444) -> (-32.0674, 37.0947) construction
  arc A147 (-32.1683, 36.6301) -> (-32.0674, 37.0947) centre (-32.4322, 36.9306) ccw
  arc A148 (-32.1683, 36.6301) -> (-32.3095, 36.5056) centre (0, 0) ccw
  arc A149 (-32.7831, 36.4638) -> (-32.3095, 36.5056) centre (-32.5746, 36.8051) ccw
  spline S74 degree 3 poles (-32.7831, 36.4638) (-33.4865, 36.8772) (-34.0155, 37.1549) (-34.6354, 37.4352) knots 0 0 0 0 1 1 1 1
  line L222 (-32.7831, 36.4638) -> (-33.4865, 36.8772) construction
  line L223 (-33.4865, 36.8772) -> (-34.0155, 37.1549) construction
  line L224 (-34.0155, 37.1549) -> (-34.6354, 37.4352) construction
  arc A150 (-34.6354, 37.4352) -> (-35.1866, 36.9176) centre (0, 0) ccw
  spline S75 degree 3 poles (-35.1866, 36.9176) (-34.9457, 36.2814) (-34.7018, 35.7359) (-34.3334, 35.008) knots 0 0 0 0 1 1 1 1
  line L225 (-35.1866, 36.9176) -> (-34.9457, 36.2814) construction
  line L226 (-34.9457, 36.2814) -> (-34.7018, 35.7359) construction
  line L227 (-34.7018, 35.7359) -> (-34.3334, 35.008) construction
  arc A151 (-34.4048, 34.538) -> (-34.3334, 35.008) centre (-34.6871, 34.8213) ccw
  arc A152 (-34.4048, 34.538) -> (-34.538, 34.4048) centre (0, 0) ccw
  arc A153 (-35.008, 34.3334) -> (-34.538, 34.4048) centre (-34.8213, 34.6871) ccw
  spline S76 degree 3 poles (-35.008, 34.3334) (-35.7359, 34.7018) (-36.2814, 34.9457) (-36.9176, 35.1866) knots 0 0 0 0 1 1 1 1
  line L228 (-35.008, 34.3334) -> (-35.7359, 34.7018) construction
  line L229 (-35.7359, 34.7018) -> (-36.2814, 34.9457) construction
  line L230 (-36.2814, 34.9457) -> (-36.9176, 35.1866) construction
  arc A154 (-36.9176, 35.1866) -> (-37.4352, 34.6354) centre (0, 0) ccw
  spline S77 degree 3 poles (-37.4352, 34.6354) (-37.1549, 34.0155) (-36.8772, 33.4865) (-36.4638, 32.7831) knots 0 0 0 0 1 1 1 1
  line L231 (-37.4352, 34.6354) -> (-37.1549, 34.0155) construction
  line L232 (-37.1549, 34.0155) -> (-36.8772, 33.4865) construction
  line L233 (-36.8772, 33.4865) -> (-36.4638, 32.7831) construction
  arc A155 (-36.5056, 32.3095) -> (-36.4638, 32.7831) centre (-36.8051, 32.5746) ccw
  arc A156 (-36.5056, 32.3095) -> (-36.6301, 32.1683) centre (0, 0) ccw
  arc A157 (-37.0947, 32.0674) -> (-36.6301, 32.1683) centre (-36.9306, 32.4322) ccw
  spline S78 degree 3 poles (-37.0947, 32.0674) (-37.8444, 32.3894) (-38.404, 32.5986) (-39.0542, 32.7991) knots 0 0 0 0 1 1 1 1
  line L234 (-37.0947, 32.0674) -> (-37.8444, 32.3894) construction
  line L235 (-37.8444, 32.3894) -> (-38.404, 32.5986) construction
  line L236 (-38.404, 32.5986) -> (-39.0542, 32.7991) construction
  arc A158 (-39.0542, 32.7991) -> (-39.5361, 32.2165) centre (0, 0) ccw
  spline S79 degree 3 poles (-39.5361, 32.2165) (-39.2174, 31.6154) (-38.9071, 31.1049) (-38.4503, 30.4288) knots 0 0 0 0 1 1 1 1
  line L237 (-39.5361, 32.2165) -> (-39.2174, 31.6154) construction
  line L238 (-39.2174, 31.6154) -> (-38.9071, 31.1049) construction
  line L239 (-38.9071, 31.1049) -> (-38.4503, 30.4288) construction
  arc A159 (-38.4623, 29.9535) -> (-38.4503, 30.4288) centre (-38.7779, 30.1993) ccw
  arc A160 (-38.4623, 29.9535) -> (-38.5777, 29.8048) centre (0, 0) ccw
  arc A161 (-39.0351, 29.675) -> (-38.5777, 29.8048) centre (-38.8942, 30.0493) ccw
  spline S80 degree 3 poles (-39.0351, 29.675) (-39.8034, 29.9493) (-40.3751, 30.1229) (-41.0366, 30.2821) knots 0 0 0 0 1 1 1 1
  line L240 (-39.0351, 29.675) -> (-39.8034, 29.9493) construction
  line L241 (-39.8034, 29.9493) -> (-40.3751, 30.1229) construction
  line L242 (-40.3751, 30.1229) -> (-41.0366, 30.2821) construction
  arc A162 (-41.0366, 30.2821) -> (-41.481, 29.6704) centre (0, 0) ccw
  spline S81 degree 3 poles (-41.481, 29.6704) (-41.1252, 29.0905) (-40.7834, 28.6005) (-40.2851, 27.9545) knots 0 0 0 0 1 1 1 1
  line L243 (-41.481, 29.6704) -> (-41.1252, 29.0905) construction
  line L244 (-41.1252, 29.0905) -> (-40.7834, 28.6005) construction
  line L245 (-40.7834, 28.6005) -> (-40.2851, 27.9545) construction
  arc A163 (-40.2672, 27.4794) -> (-40.2851, 27.9545) centre (-40.5976, 27.7048) ccw
  arc A164 (-40.2672, 27.4794) -> (-40.373, 27.3237) centre (0, 0) ccw
  arc A165 (-40.8213, 27.1654) -> (-40.373, 27.3237) centre (-40.7043, 27.5479) ccw
  spline S82 degree 3 poles (-40.8213, 27.1654) (-41.6054, 27.3909) (-42.1869, 27.5283) (-42.857, 27.6457) knots 0 0 0 0 1 1 1 1
  line L246 (-40.8213, 27.1654) -> (-41.6054, 27.3909) construction
  line L247 (-41.6054, 27.3909) -> (-42.1869, 27.5283) construction
  line L248 (-42.1869, 27.5283) -> (-42.857, 27.6457) construction
  arc A166 (-42.857, 27.6457) -> (-43.2622, 27.0072) centre (0, 0) ccw
  spline S83 degree 3 poles (-43.2622, 27.0072) (-42.8706, 26.4509) (-42.4987, 25.9832) (-41.9609, 25.3698) knots 0 0 0 0 1 1 1 1
  line L249 (-43.2622, 27.0072) -> (-42.8706, 26.4509) construction
  line L250 (-42.8706, 26.4509) -> (-42.4987, 25.9832) construction
  line L251 (-42.4987, 25.9832) -> (-41.9609, 25.3698) construction
  arc A167 (-41.9132, 24.8967) -> (-41.9609, 25.3698) centre (-42.2571, 25.101) ccw
  arc A168 (-41.9132, 24.8967) -> (-42.009, 24.7347) centre (0, 0) ccw
  arc A169 (-42.4465, 24.5486) -> (-42.009, 24.7347) centre (-42.3537, 24.9377) ccw
  spline S84 degree 3 poles (-42.4465, 24.5486) (-43.2432, 24.7244) (-43.8322, 24.825) (-44.5083, 24.9001) knots 0 0 0 0 1 1 1 1
  line L252 (-42.4465, 24.5486) -> (-43.2432, 24.7244) construction
  line L253 (-43.2432, 24.7244) -> (-43.8322, 24.825) construction
  line L254 (-43.8322, 24.825) -> (-44.5083, 24.9001) construction
  arc A170 (-44.5083, 24.9001) -> (-44.8726, 24.2375) centre (0, 0) ccw
  spline S85 degree 3 poles (-44.8726, 24.2375) (-44.4469, 23.7068) (-44.0464, 23.2635) (-43.471, 22.685) knots 0 0 0 0 1 1 1 1
  line L255 (-44.8726, 24.2375) -> (-44.4469, 23.7068) construction
  line L256 (-44.4469, 23.7068) -> (-44.0464, 23.2635) construction
  line L257 (-44.0464, 23.2635) -> (-43.471, 22.685) construction
  arc A171 (-43.3938, 22.2159) -> (-43.471, 22.685) centre (-43.7498, 22.3981) ccw
  arc A172 (-43.3938, 22.2159) -> (-43.4792, 22.0481) centre (0, 0) ccw
  arc A173 (-43.9042, 21.8349) -> (-43.4792, 22.0481) centre (-43.836, 22.229) ccw
  spline S86 degree 3 poles (-43.9042, 21.8349) (-44.7103, 21.9604) (-45.3044, 22.0238) (-45.984, 22.0563) knots 0 0 0 0 1 1 1 1
  line L258 (-43.9042, 21.8349) -> (-44.7103, 21.9604) construction
  line L259 (-44.7103, 21.9604) -> (-45.3044, 22.0238) construction
  line L260 (-45.3044, 22.0238) -> (-45.984, 22.0563) construction
  arc A174 (-45.984, 22.0563) -> (-46.3059, 21.3721) centre (0, 0) ccw
  spline S87 degree 3 poles (-46.3059, 21.3721) (-45.8478, 20.8692) (-45.4202, 20.4519) (-44.8097, 19.9107) knots 0 0 0 0 1 1 1 1
  line L261 (-46.3059, 21.3721) -> (-45.8478, 20.8692) construction
  line L262 (-45.8478, 20.8692) -> (-45.4202, 20.4519) construction
  line L263 (-45.4202, 20.4519) -> (-44.8097, 19.9107) construction
  arc A175 (-44.7031, 19.4473) -> (-44.8097, 19.9107) centre (-45.0699, 19.6069) ccw
  arc A176 (-44.7031, 19.4473) -> (-44.7778, 19.2745) centre (0, 0) ccw
  arc A177 (-45.1886, 19.035) -> (-44.7778, 19.2745) centre (-45.1452, 19.4327) ccw
  spline S88 degree 3 poles (-45.1886, 19.035) (-46.001, 19.1096) (-46.5979, 19.1356) (-47.2782, 19.1254) knots 0 0 0 0 1 1 1 1
  line L264 (-45.1886, 19.035) -> (-46.001, 19.1096) construction
  line L265 (-46.001, 19.1096) -> (-46.5979, 19.1356) construction
  line L266 (-46.5979, 19.1356) -> (-47.2782, 19.1254) construction
  arc A178 (-47.2782, 19.1254) -> (-47.5565, 18.4224) centre (0, 0) ccw
  spline S89 degree 3 poles (-47.5565, 18.4224) (-47.0677, 17.9492) (-46.6147, 17.5595) (-45.9714, 17.0578) knots 0 0 0 0 1 1 1 1
  line L267 (-47.5565, 18.4224) -> (-47.0677, 17.9492) construction
  line L268 (-47.0677, 17.9492) -> (-46.6147, 17.5595) construction
  line L269 (-46.6147, 17.5595) -> (-45.9714, 17.0578) construction
  arc A179 (-45.836, 16.602) -> (-45.9714, 17.0578) centre (-46.2121, 16.7382) ccw
  arc A180 (-45.836, 16.602) -> (-45.8997, 16.4249) centre (0, 0) ccw
  arc A181 (-46.2946, 16.1601) -> (-45.8997, 16.4249) centre (-46.2763, 16.5596) ccw
  spline S90 degree 3 poles (-46.2946, 16.1601) (-47.1102, 16.1835) (-47.7075, 16.172) (-48.3858, 16.119) knots 0 0 0 0 1 1 1 1
  line L270 (-46.2946, 16.1601) -> (-47.1102, 16.1835) construction
  line L271 (-47.1102, 16.1835) -> (-47.7075, 16.172) construction
  line L272 (-47.7075, 16.172) -> (-48.3858, 16.119) construction
  arc A182 (-48.3858, 16.119) -> (-48.6194, 15.3999) centre (0, 0) ccw
  spline S91 degree 3 poles (-48.6194, 15.3999) (-48.1018, 14.9584) (-47.6253, 14.5979) (-46.9518, 14.1375) knots 0 0 0 0 1 1 1 1
  line L273 (-48.6194, 15.3999) -> (-48.1018, 14.9584) construction
  line L274 (-48.1018, 14.9584) -> (-47.6253, 14.5979) construction
  line L275 (-47.6253, 14.5979) -> (-46.9518, 14.1375) construction
  arc A183 (-46.788, 13.6912) -> (-46.9518, 14.1375) centre (-47.1719, 13.8035) ccw
  arc A184 (-46.788, 13.6912) -> (-46.8405, 13.5104) centre (0, 0) ccw
  arc A185 (-47.218, 13.2213) -> (-46.8405, 13.5104) centre (-47.2248, 13.6213) ccw
  spline S92 degree 3 poles (-47.218, 13.2213) (-48.0334, 13.1935) (-48.6288, 13.1445) (-49.3024, 13.049) knots 0 0 0 0 1 1 1 1
  line L276 (-47.218, 13.2213) -> (-48.0334, 13.1935) construction
  line L277 (-48.0334, 13.1935) -> (-48.6288, 13.1445) construction
  line L278 (-48.6288, 13.1445) -> (-49.3024, 13.049) construction
  arc A186 (-49.3024, 13.049) -> (-49.4905, 12.3167) centre (0, 0) ccw
  spline S93 degree 3 poles (-49.4905, 12.3167) (-48.9462, 11.9085) (-48.448, 11.5787) (-47.7468, 11.1615) knots 0 0 0 0 1 1 1 1
  line L279 (-49.4905, 12.3167) -> (-48.9462, 11.9085) construction
  line L280 (-48.9462, 11.9085) -> (-48.448, 11.5787) construction
  line L281 (-48.448, 11.5787) -> (-47.7468, 11.1615) construction
  arc A187 (-47.5553, 10.7263) -> (-47.7468, 11.1615) centre (-47.9455, 10.8143) ccw
  arc A188 (-47.5553, 10.7263) -> (-47.5964, 10.5426) centre (0, 0) ccw
  arc A189 (-47.955, 10.2304) -> (-47.5964, 10.5426) centre (-47.9869, 10.6291) ccw
  spline S94 degree 3 poles (-47.955, 10.2304) (-48.767, 10.1514) (-49.3582, 10.0651) (-50.0245, 9.9276) knots 0 0 0 0 1 1 1 1
  line L282 (-47.955, 10.2304) -> (-48.767, 10.1514) construction
  line L283 (-48.767, 10.1514) -> (-49.3582, 10.0651) construction
  line L284 (-49.3582, 10.0651) -> (-50.0245, 9.9276) construction
  arc A190 (-50.0245, 9.9276) -> (-50.1662, 9.1848) centre (0, 0) ccw
  spline S95 degree 3 poles (-50.1662, 9.1848) (-49.5973, 8.8117) (-49.0794, 8.5138) (-48.3535, 8.1414) knots 0 0 0 0 1 1 1 1
  line L285 (-50.1662, 9.1848) -> (-49.5973, 8.8117) construction
  line L286 (-49.5973, 8.8117) -> (-49.0794, 8.5138) construction
  line L287 (-49.0794, 8.5138) -> (-48.3535, 8.1414) construction
  arc A191 (-48.135, 7.7191) -> (-48.3535, 8.1414) centre (-48.5299, 7.7825) ccw
  arc A192 (-48.135, 7.7191) -> (-48.1644, 7.5332) centre (0, 0) ccw
  arc A193 (-48.5027, 7.1991) -> (-48.1644, 7.5332) centre (-48.5596, 7.595) ccw
  spline S96 degree 3 poles (-48.5027, 7.1991) (-49.3082, 7.0693) (-49.8928, 6.946) (-50.5492, 6.7669) knots 0 0 0 0 1 1 1 1
  line L288 (-48.5027, 7.1991) -> (-49.3082, 7.0693) construction
  line L289 (-49.3082, 7.0693) -> (-49.8928, 6.946) construction
  line L290 (-49.8928, 6.946) -> (-50.5492, 6.7669) construction
  arc A194 (-50.5492, 6.7669) -> (-50.6439, 6.0168) centre (0, 0) ccw
  spline S97 degree 3 poles (-50.6439, 6.0168) (-50.0527, 5.68) (-49.5171, 5.4153) (-48.7692, 5.0892) knots 0 0 0 0 1 1 1 1
  line L291 (-50.6439, 6.0168) -> (-50.0527, 5.68) construction
  line L292 (-50.0527, 5.68) -> (-49.5171, 5.4153) construction
  line L293 (-49.5171, 5.4153) -> (-48.7692, 5.0892) construction
  arc A195 (-48.5247, 4.6815) -> (-48.7692, 5.0892) centre (-48.9228, 4.7199) ccw
  arc A196 (-48.5247, 4.6815) -> (-48.5424, 4.4941) centre (0, 0) ccw
  arc A197 (-48.859, 4.1394) -> (-48.5424, 4.4941) centre (-48.9407, 4.5309) ccw
  spline S98 degree 3 poles (-48.859, 4.1394) (-49.6548, 3.9592) (-50.2305, 3.7995) (-50.8743, 3.5795) knots 0 0 0 0 1 1 1 1
  line L294 (-48.859, 4.1394) -> (-49.6548, 3.9592) construction
  line L295 (-49.6548, 3.9592) -> (-50.2305, 3.7995) construction
  line L296 (-50.2305, 3.7995) -> (-50.8743, 3.5795) construction
  arc A198 (-50.8743, 3.5795) -> (-50.9218, 2.8249) centre (0, 0) ccw
  spline S99 degree 3 poles (-50.9218, 2.8249) (-50.3106, 2.526) (-49.7595, 2.2954) (-48.9926, 2.0169) knots 0 0 0 0 1 1 1 1
  line L297 (-50.9218, 2.8249) -> (-50.3106, 2.526) construction
  line L298 (-50.3106, 2.526) -> (-49.7595, 2.2954) construction
  line L299 (-49.7595, 2.2954) -> (-48.9926, 2.0169) construction
  arc A199 (-48.7229, 1.6254) -> (-48.9926, 2.0169) centre (-49.1227, 1.6387) ccw
  arc A200 (-48.7229, 1.6254) -> (-48.7288, 1.4372) centre (0, 0) ccw
  arc A201 (-49.0225, 1.0633) -> (-48.7288, 1.4372) centre (-49.1286, 1.449) ccw
  spline S100 degree 3 poles (-49.0225, 1.0633) (-49.8054, 0.8336) (-50.3699, 0.638) (-50.9987, 0.3781) knots 0 0 0 0 1 1 1 1
  line L300 (-49.0225, 1.0633) -> (-49.8054, 0.8336) construction
  line L301 (-49.8054, 0.8336) -> (-50.3699, 0.638) construction
  line L302 (-50.3699, 0.638) -> (-50.9987, 0.3781) construction
  arc A202 (-50.9987, 0.3781) -> (-50.9987, -0.3781) centre (0, 0) ccw
  spline S101 degree 3 poles (-50.9987, -0.3781) (-50.3699, -0.638) (-49.8054, -0.8336) (-49.0225, -1.0633) knots 0 0 0 0 1 1 1 1
  line L303 (-50.9987, -0.3781) -> (-50.3699, -0.638) construction
  line L304 (-50.3699, -0.638) -> (-49.8054, -0.8336) construction
  line L305 (-49.8054, -0.8336) -> (-49.0225, -1.0633) construction
  arc A203 (-48.7288, -1.4372) -> (-49.0225, -1.0633) centre (-49.1286, -1.449) ccw
  arc A204 (-48.7288, -1.4372) -> (-48.7229, -1.6254) centre (0, 0) ccw
  arc A205 (-48.9926, -2.0169) -> (-48.7229, -1.6254) centre (-49.1227, -1.6387) ccw
  spline S102 degree 3 poles (-48.9926, -2.0169) (-49.7595, -2.2954) (-50.3106, -2.526) (-50.9218, -2.8249) knots 0 0 0 0 1 1 1 1
  line L306 (-48.9926, -2.0169) -> (-49.7595, -2.2954) construction
  line L307 (-49.7595, -2.2954) -> (-50.3106, -2.526) construction
  line L308 (-50.3106, -2.526) -> (-50.9218, -2.8249) construction
  arc A206 (-50.9218, -2.8249) -> (-50.8743, -3.5795) centre (0, 0) ccw
  spline S103 degree 3 poles (-50.8743, -3.5795) (-50.2305, -3.7995) (-49.6548, -3.9592) (-48.859, -4.1394) knots 0 0 0 0 1 1 1 1
  line L309 (-50.8743, -3.5795) -> (-50.2305, -3.7995) construction
  line L310 (-50.2305, -3.7995) -> (-49.6548, -3.9592) construction
  line L311 (-49.6548, -3.9592) -> (-48.859, -4.1394) construction
  arc A207 (-48.5424, -4.4941) -> (-48.859, -4.1394) centre (-48.9407, -4.5309) ccw